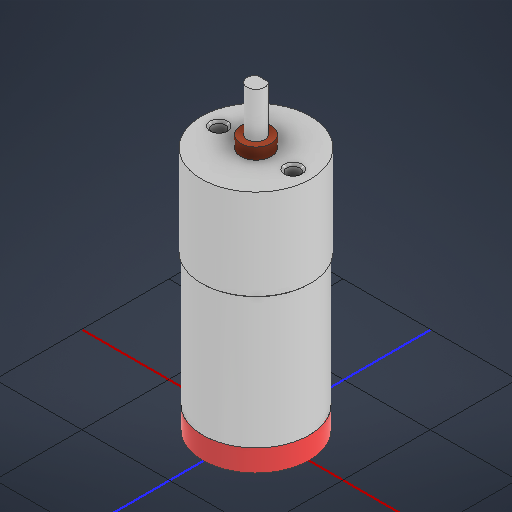
# Autodesk Inventor part: dc12v1200rpm
Saved by Autodesk Inventor 2027 (Build 310192000, 192)
## iProperties
Created: 2026-05-11
Part Number: dc12v1200rpm
Material: Generic
Document SubType Name: Modeling
Designer: maksi
Density: 1 g/cm^3
Appearance: Aluminum - Polished
Author: maksi
Autodesk Inventor part; units mm, degrees
ref_plane "YZ Plane" through (0, 0, 0) normal (1, 0, 0) x (0, 1, 0)
ref_plane "XZ Plane" through (0, 0, 0) normal (0, 1, 0) x (-1, 0, 0)
ref_plane "XY Plane" through (0, 0, 0) normal (0, 0, 1) x (1, 0, 0)
sketch "Sketch1" plane through (0, 0, 0) normal (0, 1, 0) x (-1, 0, 0)
  circle A0 centre (0, 0) radius 12.2
  dimension "d0" = 24.4
  constraints: 1 centre point, 1 coincident
  measures "d0" diameter of A0
extrude "Extrusion1" add sketch "Sketch1" along normal blind 30.1
sketch "Sketch2" plane through (0, 30.1, 0) normal (0, 1, 0) x (1, 0, 0)
  circle A0 centre (0, 0) radius 12.5
  dimension "d3" = 25
  constraints: 1 centre point, 1 coincident
  measures "d3" diameter of A0
extrude "Extrusion2" add sketch "Sketch2" along normal blind 21 separate body
chamfer "Chamfer1" distance 0.25 angle 45 1 edges at (-12.5, 30.1, 0)
sketch "Sketch3" plane through (0, 51.1, 0) normal (0, 1, 0) x (1, 0, 0)
  circle A0 centre (0, 0) radius 8.55
  point P0 (-8.55, 0)
  point P1 (8.55, 0)
  dimension "d9" = 17.1
  constraints: 2 point on circle, 1 centre point, 1 coincident
  measures "d9" diameter of A0
hole "Hole1" at (-8.55, 51.1, 0) at (8.55, 51.1, 0) direction (0, -1, 0) diameter 3 depth 12 tip angle 118 countersink diameter 4 countersink angle 90 bodies 2
sketch "Sketch4" plane through (0, 51.1, 0) normal (0, 1, 0) x (1, 0, 0)
  circle A0 centre (0, 0) radius 3.5
  circle A1 centre (0, 0) radius 2
  dimension "d18" = 7
  dimension "d19" = 4
  constraints: 2 centre point, 2 coincident
  measures "d18" diameter of A0
  measures "d19" diameter of A1
extrude "Extrusion3" add sketch "Sketch4" along normal blind 2.6 separate body contours A0 | A1
extrude "Extrusion4" add sketch "Sketch4" along normal blind 10.4 from surface at 2.6 separate body contours A1
sketch "Sketch5" plane through (0, 64.1, 0) normal (0, 1, 0) x (1, 0, 0)
  circle A0 centre (0, 0) radius 2 projected
  line L0 (0, 0) -> (0, 1.5) construction
  line L1 (0, 1.5) -> (1.3229, 1.5) construction
  line L2 (0, 1.5) -> (-1.3229, 1.5) construction
  line L3 (-1.3229, 1.5) -> (1.3229, 1.5)
  dimension "d24" = 1.5
  constraints: 8 end point, 2 point on circle, 1 horizontal, 1 perpendicular, 1 point on line, 1 vertical
  measures "d24" distance of L0.start L0.end
extrude "Extrusion5" cut sketch "Sketch5" against normal up to surface (10.4 mm away) contours L3 A0 picked at (-0.3089, 1.5908) bodies 4
sketch "Sketch6" plane through (0, 0, 0) normal (0, -1, 0) x (1, 0, 0)
  circle A0 centre (0, 0) radius 12.2 projected
extrude "Extrusion6" add sketch "Sketch6" along normal blind 5 from surface at 0 separate body
body "Solid1"
body "Solid2"
body "Solid3"
body "Solid4"
body "Solid6"
